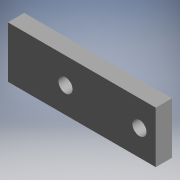
# Autodesk Inventor part: rollerHolderInnerZ
Saved by Autodesk Inventor 2019 (Build 230136000, 136)
## iProperties
Created: 2019-05-13
Part Number: rollerHolderInnerZ
Material: Generic
Document SubType Name: Modeling
Designer: Alex Jones
Density: 1 g/cm^3
Appearance: Default
Author: Alex Jones
Autodesk Inventor part; units mm, degrees
ref_plane "YZ Plane" through (0, 0, 0) normal (1, 0, 0) x (0, 1, 0)
ref_plane "XZ Plane" through (0, 0, 0) normal (0, 1, 0) x (-1, 0, 0)
ref_plane "XY Plane" through (0, 0, 0) normal (0, 0, 1) x (1, 0, 0)
sketch "Sketch1" plane through (0, 0, 0) normal (0, 0, 1) x (1, 0, 0)
  line L0 (0, -12.35) -> (-250, -12.35) projected
  line L1 (0, -12.35) -> (0, -7.2) projected
  line L2 (0, -7.2) -> (-250, -7.2) projected
  line L3 (-250, -12.35) -> (-250, -7.2) projected
  line L4 (-250, 5.15) -> (0, 5.15) projected
  line L5 (-250, 0) -> (-250, 5.15) projected
  line L6 (0, 0) -> (-250, 0) projected
  line L7 (0, 0) -> (0, 5.15) projected
  line L8 (0, 6.4) -> (-250, 6.4) projected
  line L9 (-250, -13.6) -> (0, -13.6) projected
  line L10 (-159.051, -15.85) -> (90.949, -15.85) projected
  line L11 (-159.051, -21) -> (-159.051, -15.85) projected
  line L12 (90.949, -21) -> (-159.051, -21) projected
  line L13 (90.949, -21) -> (90.949, -15.85) projected
  line L14 (90.949, 8.65) -> (-159.051, 8.65) projected
  line L15 (90.949, 13.8) -> (90.949, 8.65) projected
  line L16 (-159.051, 13.8) -> (90.949, 13.8) projected
  line L17 (-159.051, 13.8) -> (-159.051, 8.65) projected
  line L18 (-159.051, 7.4) -> (90.949, 7.4) projected
  line L19 (90.949, -14.6) -> (-159.051, -14.6) projected
  line L20 (-159.051, -34.6) -> (90.949, -34.6) projected
  line L21 (90.949, 27.4) -> (-159.051, 27.4) projected
  line L22 (-50.9068, -42.05) -> (-6.1068, -42.05) projected
  line L23 (-6.1068, -42.05) -> (-6.1068, -35.7) projected
  line L24 (-50.9068, -35.7) -> (-6.1068, -35.7) projected
  line L25 (-50.9068, -42.05) -> (-50.9068, -35.7) projected
  line L26 (-50.9068, 28.5) -> (-6.1068, 28.5) projected
  line L27 (-6.1068, 28.5) -> (-6.1068, 34.85) projected
  line L28 (-50.9068, 34.85) -> (-6.1068, 34.85) projected
  line L29 (-50.9068, 28.5) -> (-50.9068, 34.85) projected
  line L30 (-50.9068, -42.05) -> (-50.9068, 34.85) construction
  line L31 (-6.1068, -42.05) -> (-6.1068, 34.85) construction
  line L32 (-50.9068, -13.6) -> (-6.1068, -13.6)
  line L33 (-6.1068, 6.4) -> (-50.9068, 6.4)
  line L34 (-50.9068, 6.4) -> (-50.9068, -13.6)
  line L35 (-6.1068, -13.6) -> (6.5932, -13.6)
  line L36 (6.5932, -13.6) -> (6.5932, 6.4)
  line L37 (6.5932, 6.4) -> (-6.1068, 6.4)
  line L38 (-28.5068, -35.7) -> (-28.5068, 28.5) construction
  line L39 (6.5932, -13.6) -> (-6.1068, 6.4) construction
  circle A0 centre (0.2432, -3.6) radius 2.75
  circle A1 centre (-28.5068, -3.6) radius 2.75
  line L40 (6.5932, 6.4) -> (-50.9068, 6.4)
  line L41 (-50.9068, 6.4) -> (-50.9068, -13.6)
  line L42 (-50.9068, -13.6) -> (6.5932, -13.6)
  line L43 (6.5932, -13.6) -> (6.5932, 6.4)
  dimension "d0" = 12.7
  dimension "d1" = 5.5
  constraints: 28 end point, 4 midpoint, 4 parallel, 4 perpendicular, 4 point on line, 3 horizontal, 2 centre point, 1 equal radius
  measures "d0" distance of L36.end L37.end
  measures "d1" diameter of A1
extrude "Extrusion1" add sketch "Sketch1" along normal blind 6.35 contours L1 L2 L34 L6 L7 L4 L8 L37 L36 L35 L9 L0 | L0 L34 L2 L1 | L34 L4 L7 L6
sketch "Sketch2" plane through (0, 0, 6.35) normal (0, 0, 1) x (1, 0, 0)
  line L0 (-50.9068, -13.6) -> (6.5932, -13.6) projected
  line L1 (6.5932, -13.6) -> (6.5932, 6.4) projected
  line L2 (-50.9068, -13.6) -> (6.5932, -13.6)
  line L3 (6.5932, -13.6) -> (6.5932, -9.79)
  line L4 (6.5932, -9.79) -> (-50.9068, -9.79)
  line L5 (-50.9068, -9.79) -> (-50.9068, -13.6)
  line L6 (6.5932, 6.4) -> (-50.9068, 6.4) projected
  line L7 (-50.9068, 6.4) -> (6.5932, 6.4)
  line L8 (6.5932, 6.4) -> (6.5932, 2.59)
  line L9 (6.5932, 2.59) -> (-50.9068, 2.59)
  line L10 (-50.9068, 2.59) -> (-50.9068, 6.4)
  point P0 (0, 0)
  dimension "d4" = 3.81
  constraints: 16 end point, 4 parallel, 2 horizontal, 2 perpendicular, 2 point on line, 1 collinear
  measures "d4" distance between parallel lines of L0 L4
ref_plane "Work Plane1" through (-50.9068, 28.5, 21.3) normal (0, 0, 1) x (1, 0, 0)
extrude "Extrusion2" add sketch "Sketch2" along normal up to surface (14.95 mm away)
sketch "Sketch3" plane through (6.5932, -13.6, 0) normal (1, 0, 0) x (0, 0, -1)
  line L0 (-21.3, 16.19) -> (-21.3, 20) projected
  line L1 (0, 0) -> (-21.3, 0)
  line L2 (-21.3, 0) -> (-21.3, 20)
  line L3 (-21.3, 20) -> (0, 20)
  line L4 (0, 20) -> (0, 0)
  point P0 (0, 13.6)
  constraints: 8 end point, 2 parallel, 1 horizontal, 1 perpendicular
extrude "Extrusion3" add sketch "Sketch3" along normal blind 6.35
sketch "Sketch5" plane through (-50.9068, -13.6, 0) normal (-1, 0, 0) x (0, 0, 1)
  line L0 (21.3, 0) -> (0, 0) projected
  line L1 (21.3, 20) -> (21.3, 0) projected
  line L2 (0, 0) -> (21.3, 0)
  line L3 (21.3, 0) -> (21.3, 20)
  line L4 (21.3, 20) -> (0, 20)
  line L5 (0, 20) -> (0, 0)
  point P0 (0, 13.6)
  constraints: 8 end point, 2 parallel, 1 horizontal, 1 perpendicular
extrude "Extrusion4" add sketch "Sketch5" against normal blind 3.81
sketch "Sketch6" plane through (-50.9068, -13.6, 0) normal (0, -1, 0) x (1, 0, 0)
  circle A0 centre (9.9, 11.4) radius 2.5 projected
  circle A1 centre (34.9, 11.4) radius 2.5 projected
  point P0 (50.9068, 0)
extrude "Extrusion5" cut sketch "Sketch6" against normal through all
body "Solid1"
